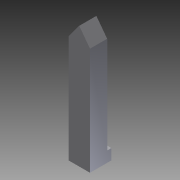
# Autodesk Inventor part: Needle
Saved by Autodesk Inventor 2012 (Build 160160000, 160)
## iProperties
Created: 2011-08-19
Part Number: Needle
Material: Default
Document SubType Name: Modeling
Designer: Minh Tran
Density: 1 g/cm^3
Author: Minh Tran
Autodesk Inventor part; units mm, degrees
ref_plane "YZ Plane" through (0, 0, 0) normal (1, 0, 0) x (0, 1, 0)
ref_plane "XZ Plane" through (0, 0, 0) normal (0, 1, 0) x (-1, 0, 0)
ref_plane "XY Plane" through (0, 0, 0) normal (0, 0, 1) x (1, 0, 0)
sketch "Sketch1" plane through (0, 0, 0) normal (0, 0, 1) x (1, 0, 0)
  line L0 (6.3387, 0) -> (6.3387, 31.7461)
  line L1 (0, 31.7461) -> (3.15, 36.0063)
  line L2 (3.15, 36.0063) -> (6.3387, 31.7461)
  line L3 (6.3387, 0) -> (0, 0)
  line L4 (0, 0) -> (0, 31.7461)
  constraints: 10 end point, 2 perpendicular, 1 vertical
extrude "Extrusion1" add sketch "Sketch1" along normal blind 5.08
sketch "Sketch2" plane through (0, 0, 0) normal (0, 0, -1) x (-1, 0, 0)
  line L0 (0, 0) -> (-6.3387, 0) projected
  line L1 (0, 31.7461) -> (0, 0) projected
  line L2 (-6.3387, 0) -> (0, 0)
  line L3 (0, 0) -> (0, 3.1419)
  line L4 (0, 3.1419) -> (-6.3387, 3.1419)
  line L5 (-6.3387, 3.1419) -> (-6.3387, 0)
  constraints: 8 end point, 2 parallel, 1 horizontal, 1 perpendicular, 1 point on line
extrude "Extrusion2" add sketch "Sketch2" along normal blind 1.27
body "Solid1"
